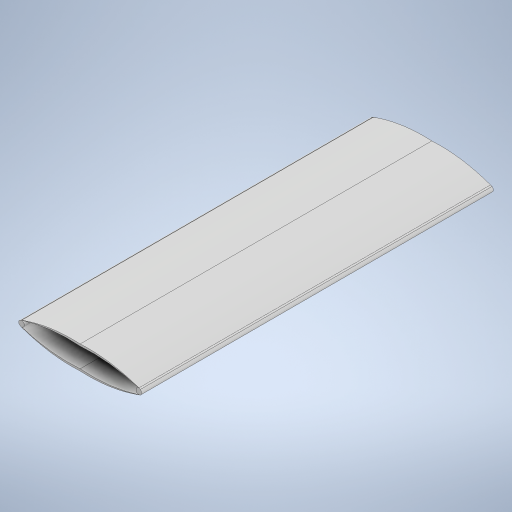
# Autodesk Inventor part: Conveyer
Saved by Autodesk Inventor 2024 (Build 280153000, 153)
## iProperties
Created: 2024-09-09
Part Number: Conveyer
Material: Generic
Document SubType Name: Modeling
Designer: srira
Density: 1 g/cm^3
Appearance: Default
Author: srira
Autodesk Inventor part; units mm, degrees
ref_plane "YZ Plane" through (0, 0, 0) normal (1, 0, 0) x (0, 1, 0)
ref_plane "XZ Plane" through (0, 0, 0) normal (0, 1, 0) x (-1, 0, 0)
ref_plane "XY Plane" through (0, 0, 0) normal (0, 0, 1) x (1, 0, 0)
sketch "Sketch1" plane through (0, 0, 0) normal (0, 0, 1) x (1, 0, 0)
  circle A0 centre (-150, 0) radius 7.5
  arc A1 (0, 25) -> (-150, 7.5) centre (-30.4951, -365.2208) ccw
  line L0 (-33.8172, 0) -> (-25.2797, 0)
  arc A2 (-150, -7.5) -> (0, -25) centre (-30.4951, 365.2208) ccw
  line L1 (0, 7.5) -> (0, -7.5)
  circle A3 centre (150, 0) radius 7.5
  arc A4 (150, 7.5) -> (0, 25) centre (30.4951, -365.2208) ccw
  arc A5 (0, -25) -> (150, -7.5) centre (30.4951, 365.2208) ccw
  arc A6 (-156.6413, 5.305) -> (-156.6413, -5.305) centre (-150, 0) ccw
  arc A7 (0, 30.1071) -> (-156.6413, 5.305) centre (-20.4803, -347.5929) ccw
  arc A8 (-156.6413, -5.305) -> (0, -30.1071) centre (-20.4803, 347.5929) ccw
  arc A9 (156.6413, 5.305) -> (0, 30.1071) centre (20.4803, -347.5929) ccw
  arc A10 (0, -30.1071) -> (156.6413, -5.305) centre (20.4803, 347.5929) ccw
  point P0 (0, 0)
  point P1 (150, -7.5)
  point P2 (-150, -7.5)
  point P3 (-150.9875, -7.4347)
  point P4 (154.1184, -6.2681)
  point P5 (154.1184, 6.2681)
  point P6 (-150.9875, 7.4347)
  dimension "d0" = 15
  dimension "d1" = 17
  constraints: 20 point on circle, 14 symmetric about line, 9 centre point, 4 end point, 2 vertical, 1 coincident, 1 horizontal, 12 other
  measures "d1" diameter of A6
extrude "Extrusion1" add sketch "Sketch1" along normal blind 900 contours A0 A8 A7 | A0 A7 A9 A3 A4 A1 | A2 A5 A3 A10 A8 A0 | A7 A0 | A0 A8 | A3 A9 A10
body "Solid1"
